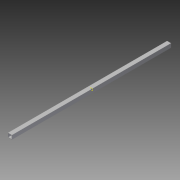
# Autodesk Inventor part: FE-00036Support
Saved by Autodesk Inventor 2013 (Build 170138000, 138)
## iProperties
Created: 2013-01-14
Part Number: FE-00036Support
Material: Steel
Document SubType Name: Modeling
Designer: Phillip
Density: 1 g/cm^3
d0: 70.350 in
d1: 0.00 deg
Author: Phillip
Autodesk Inventor part; units mm, degrees
ref_plane "YZ Plane" through (0, 0, 0) normal (1, 0, 0) x (0, 1, 0)
ref_plane "XZ Plane" through (0, 0, 0) normal (0, 1, 0) x (-1, 0, 0)
ref_plane "XY Plane" through (0, 0, 0) normal (0, 0, 1) x (1, 0, 0)
sketch "Sketch1" plane through (0, 0, 0) normal (0, 0, 1) x (1, 0, 0)
  line L0 (44.45, -44.45) -> (44.45, 0)
  line L1 (44.45, 0) -> (0, 0)
  line L2 (0, 0) -> (0, -44.45)
  line L3 (0, -44.45) -> (44.45, -44.45)
  line L4 (41.275, -41.275) -> (41.275, -3.175)
  line L5 (3.175, -41.275) -> (41.275, -41.275)
  line L6 (3.175, -3.175) -> (3.175, -41.275)
  line L7 (41.275, -3.175) -> (3.175, -3.175)
  point P0 (24.7686, -16.9571)
  constraints: 16 end point
extrude "Extrusion1" add sketch "Sketch1" against normal blind 1786.89
ref_plane "Work Plane1" through (44.45, 0, -893.445) normal (0, 0, -1) x (-1, 0, 0)
body "Solid1"
